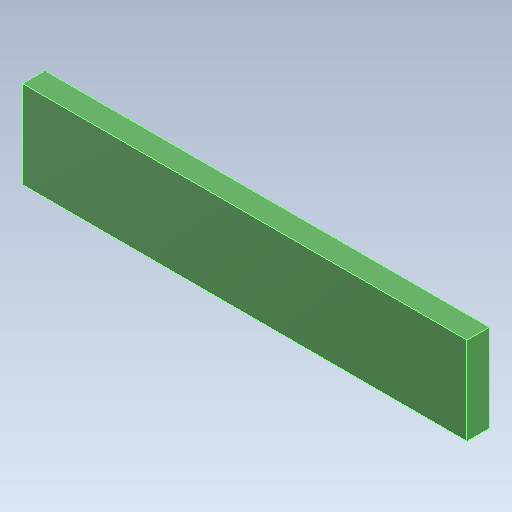
# Autodesk Inventor part: U_1___LOGO_UT_ECE
Saved by Autodesk Inventor 2021 (Build 250183000, 183)
## iProperties
Created: 2020-11-03
Part Number: U_1___LOGO_UT_ECE
Material: Generic
Document SubType Name: Modeling
Designer: faiya
Density: 1 g/cm^3
Appearance: __LOGO_UT_ECE, U_1___LOGO_UT_ECE
Author: faiya
Autodesk Inventor part; units mm, degrees
ref_plane "YZ Plane" through (0, 0, 0) normal (1, 0, 0) x (0, 1, 0)
ref_plane "XZ Plane" through (0, 0, 0) normal (0, 1, 0) x (-1, 0, 0)
ref_plane "XY Plane" through (0, 0, 0) normal (0, 0, 1) x (1, 0, 0)
sketch "__LOGO_UT_ECE, U_1___LOGO_UT_ECE_66" plane through (0, 0, 0) normal (0, 0, 1) x (1, 0, 0)
  line L0 (0, 3.9243) -> (19.9009, 3.9243)
  line L1 (19.9009, 3.9243) -> (19.9009, 0)
  line L2 (19.9009, 0) -> (0, 0)
  line L3 (0, 0) -> (0, 3.9243)
  constraints: 8 end point
extrude "Extrusion1" add sketch "__LOGO_UT_ECE, U_1___LOGO_UT_ECE_66" along normal blind 1
body "Solid1"
